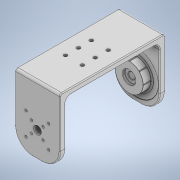
# Autodesk Inventor part: мотор_плеча_2_v2
Saved by Autodesk Inventor 2022 (Build 260153000, 153)
## iProperties
Created: 2022-12-04
Part Number: мотор_плеча_2_v2
Material: Типовые
Document SubType Name: Modeling
Designer: Папа
Density: 1 g/cm^3
Appearance: По умолчанию
Author: Папа
Autodesk Inventor part; units mm, degrees
ref_plane "YZ Plane" through (0, 0, 0) normal (1, 0, 0) x (0, 1, 0)
ref_plane "XZ Plane" through (0, 0, 0) normal (0, 1, 0) x (-1, 0, 0)
ref_plane "XY Plane" through (0, 0, 0) normal (0, 0, 1) x (1, 0, 0)
sketch "Эскиз1" plane through (0, 0, 0) normal (0, 1, 0) x (-1, 0, 0)
  line L0 (-20, -46.7) -> (20, -46.7)
  line L1 (20, -46.7) -> (20, 46.7)
  line L2 (20, 46.7) -> (-20, 46.7)
  line L3 (-20, 46.7) -> (-20, -46.7)
  line L4 (-20, -46.7) -> (20, 46.7) construction
  line L5 (20, -46.7) -> (-20, 46.7) construction
  point P0 (0, 0)
  dimension "d0" = 40
  dimension "d1" = 93.4
  constraints: 12 end point, 2 midpoint, 2 parallel, 1 horizontal, 1 perpendicular
  measures "d0" distance between parallel lines of L3 L1
  measures "d1" distance of L0.end L1.end
extrude "Выдавливание1" add sketch "Эскиз1" along normal blind 5
sketch "Эскиз5" plane through (0, 0, 0) normal (0, -1, 0) x (1, 0, 0)
  line L0 (22.9, 22.9) -> (22.9, -22.9)
  line L1 (22.9, -22.9) -> (-22.9, -22.9)
  line L2 (-22.9, -22.9) -> (-22.9, 22.9)
  line L3 (-22.9, 22.9) -> (22.9, 22.9)
  circle A0 centre (0, 0) radius 12.5
  dimension "d16" = 45.8
  dimension "d17" = 25
  constraints: 8 end point, 2 coincident, 1 centre point, 1 horizontal, 9 other
  measures "d16" distance of L2.end L0.start
  measures "d17" diameter of A0
extrude "Выдавливание5" [suppressed]
fillet "Сопряжение3" [suppressed]
ref_plane "РабПлоскость1" through (20, 0, 0) normal (0, 0, -1) x (-1, 0, 0)
sketch "Эскиз6" plane through (-20, 0, 46.7) normal (0, 0, 1) x (1, 0, 0)
  line L0 (40, 5) -> (42.9, 5) projected
  line L1 (40, 5) -> (0, 5)
  line L2 (0, 5) -> (0, -55)
  line L3 (0, -55) -> (40, -55)
  line L4 (40, -55) -> (40, 5)
  line L5 (0, 0) -> (40, 0) projected
  point P0 (20, 0)
  dimension "d25" = 55
  constraints: 8 end point, 2 parallel, 1 horizontal, 1 perpendicular, 1 point on line
  measures "d25" distance between parallel lines of L5 L3
extrude "Выдавливание6" add sketch "Эскиз6" against normal blind 5 contours L4 L3 L2 L5
fillet "Сопряжение4" radius 5 1 edges at (0, 0, 41.7)
fillet "Сопряжение5" radius 16 2 edges at (-20, -55, 44.2) (20, -55, 44.2)
mirror "Зеркальное отражение2" about plane through (20, 0, 0) normal (0, 0, -1) of "Выдавливание6", "Сопряжение5", "Сопряжение4"
sketch "Эскиз7" plane through (-20, 0, 41.7) normal (0, 0, -1) x (-1, 0, 0)
  line L0 (-40, -39) -> (-40, 5) projected
  line L1 (0, -39) -> (0, 5) projected
  line L2 (0, -10) -> (-40, -10)
  line L3 (-40, -10) -> (-40, -55)
  line L4 (-40, -55) -> (0, -55)
  line L5 (0, -55) -> (0, -10)
  line L6 (-24, -55) -> (-16, -55) projected
  arc A0 (-40, -39) -> (-24, -55) centre (-24, -39) ccw projected
  line L7 (-24, -55) -> (-16, -55) projected
  arc A1 (-16, -55) -> (0, -39) centre (-16, -39) ccw projected
  line L8 (0, -39) -> (0, -5) projected
  line L9 (-40, -5) -> (0, -5) projected
  line L10 (-40, -5) -> (-40, -39) projected
  circle A2 centre (-20, -32.5) radius 3.5
  line L11 (-40, -5) -> (-40, -39) projected
  line L12 (0, -10) -> (-40, -10)
  line L13 (-40, -10) -> (-40, -5)
  line L14 (-40, -5) -> (0, -5)
  line L15 (0, -5) -> (0, -10)
  line L16 (0, -55) -> (-40, -10) construction
  point P0 (-20, 0)
  dimension "d31" = 40
  dimension "d33" = 7
  dimension "d107" = 5
  constraints: 18 end point, 4 parallel, 2 horizontal, 2 midpoint, 2 perpendicular, 1 centre point, 1 collinear, 1 point on line
  measures "d31" distance of L3.end L4.end
  measures "d33" diameter of A2
  measures "d107" distance between parallel lines of L14 L2
extrude "Выдавливание7" cut sketch "Эскиз7" against normal up to surface (5 mm away) contours A2
sketch "Эскиз8" plane through (-20, -5, -41.7) normal (0, 0, 1) x (1, 0, 0)
  line L0 (40, 0) -> (40, -50)
  line L1 (40, -50) -> (0, -50)
  line L2 (0, -50) -> (0, 0)
  line L3 (24, -50) -> (16, -50) projected
  line L4 (40, 0) -> (40, -34) projected
  circle A0 centre (20, -27.5) radius 18.9
  circle A1 centre (20, -27.5) radius 14.5
  line L5 (0, 0) -> (40, 0) projected
  line L6 (0, 0) -> (40, 0)
  line L7 (40, 0) -> (40, -5)
  line L8 (40, -5) -> (0, -5)
  line L9 (0, -5) -> (0, 0)
  point P0 (20, 5)
  dimension "d36" = 37.8
  dimension "d108" = 5
  dimension "d120" = 29
  constraints: 14 end point, 3 parallel, 2 centre point, 2 coincident, 2 collinear, 1 horizontal, 1 perpendicular, 1 point on line
  measures "d36" diameter of A0
  measures "d108" distance between parallel lines of L8 L5
  measures "d120" diameter of A1
extrude "Выдавливание8" cut sketch "Эскиз8" against normal blind 0.2 contours A0
sketch "Эскиз9" plane through (0, -32.5, -41.7) normal (0, 0, 1) x (1, 0, 0)
  circle A0 centre (0, 0) radius 18.9 projected
  circle A1 centre (0, 0) radius 12.35
  point P0 (0, 32.5)
  dimension "d40" = 24.7
  constraints: 1 centre point, 1 coincident
  measures "d40" diameter of A1
extrude "Выдавливание9" add sketch "Эскиз9" along normal blind 6.9 contours A1
sketch "Эскиз10" plane through (0, -32.5, -34.8) normal (0, 0, 1) x (1, 0, 0)
  circle A0 centre (0, 0) radius 12.35 projected
  circle A1 centre (-12.35, 0) radius 0.25
  point P0 (0, 32.5)
  point P1 (-12.3475, -0.25)
  point P2 (-12.3475, 0.25)
  dimension "d44" = 0.5
  constraints: 1 centre point, 2 other
  measures "d44" diameter of A1
extrude "Выдавливание10" add sketch "Эскиз10" against normal up to surface (6.9 mm away) contours A0 A1 picked at (-12.4325, 0.0101)
fillet "Сопряжение7" radius 0.4 2 edges at (-12.3475, -32.25, -38.25) (-12.3475, -32.75, -38.25)
pattern_circular "Круговой массив1" count 8 over 360 about axis through (0, -32.5, -41.7) along (0, 0, 1) of "Сопряжение7", "Выдавливание10"
fillet "Сопряжение8" radius 0.2 66 edges at (-8.9941, -41.0216, -34.8) (-8.9095, -41.4095, -34.8) (-8.5216, -41.4941, -34.8) (-4.7261, -43.9099, -34.8) (-0.3341, -44.8854, -34.8) (0, -45.1, -34.8) (0.3341, -44.8854, -34.8) (4.7261, -43.9099, -34.8) (8.5216, -41.4941, -34.8) (8.9095, -41.4095, -34.8) (8.9941, -41.0216, -34.8) (11.4099, -37.2261, -34.8) (12.3854, -32.8341, -34.8) (12.6, -32.5, -34.8) (12.3854, -32.1659, -34.8) (11.4099, -27.7739, -34.8) (8.9941, -23.9784, -34.8) (8.9095, -23.5905, -34.8) (8.5216, -23.5059, -34.8) (4.7261, -21.0901, -34.8) (0.3341, -20.1146, -34.8) (0, -19.9, -34.8) (-0.3341, -20.1146, -34.8) (-4.7261, -21.0901, -34.8) (-8.5216, -23.5059, -34.8) (-8.9095, -23.5905, -34.8) (-8.9941, -23.9784, -34.8) (-11.4099, -27.7739, -34.8) (-12.3854, -32.1659, -34.8) (-12.6, -32.5, -34.8) (-12.3854, -32.8341, -34.8) (-11.4099, -37.2261, -34.8) (-12.3854, -32.8341, -41.7) (-12.6, -32.5, -41.7) (-12.3854, -32.1659, -41.7) (-11.4099, -27.7739, -41.7) (-8.9941, -23.9784, -41.7) (-8.9095, -23.5905, -41.7) (-8.5216, -23.5059, -41.7) (-4.7261, -21.0901, -41.7) (-0.3341, -20.1146, -41.7) (0, -19.9, -41.7) (0.3341, -20.1146, -41.7) (4.7261, -21.0901, -41.7) (8.5216, -23.5059, -41.7) (8.9095, -23.5905, -41.7) (8.9941, -23.9784, -41.7) (11.4099, -27.7739, -41.7) (12.3854, -32.1659, -41.7) (12.6, -32.5, -41.7) (12.3854, -32.8341, -41.7) (11.4099, -37.2261, -41.7) (8.9941, -41.0216, -41.7) (8.9095, -41.4095, -41.7) (8.5216, -41.4941, -41.7) (4.7261, -43.9099, -41.7) (0.3341, -44.8854, -41.7) (0, -45.1, -41.7) (-0.3341, -44.8854, -41.7) (-4.7261, -43.9099, -41.7) (-8.5216, -41.4941, -41.7) (-8.9095, -41.4095, -41.7) (-8.9941, -41.0216, -41.7) (-11.4099, -37.2261, -41.7) (-18.9, -32.5, -41.7) (-18.9, -32.5, -41.9)
fillet "Сопряжение11" radius 2 2 edges at (0, 5, -46.7) (0, 5, 46.7)
ref_plane "РабПлоскость3" through (3.7349, -5, -34.5) normal (0, 0, 1) x (1, 0, 0)
sketch "Эскиз17" plane through (-20, -5, -41.7) normal (0, 0, 1) x (1, 0, 0)
  circle A0 centre (20, -27.5) radius 14.5 projected
  circle A1 centre (20, -27.5) radius 20.9
  circle A2 centre (20, -27.5) radius 22.9
  point P0 (20, 5)
  point P1 (0, -21.4329)
  point P2 (40, -21.4329)
  dimension "d70" = 2
  constraints: 2 coincident, 1 centre point, 4 other
extrude "Выдавливание14" [suppressed]
fillet "Сопряжение14" radius 0.8 32 edges at (-20, -22, -41.7) (0, -55, -41.7) (-15.3137, -50.3137, -41.7) (0, -55, -46.7) (-20, -18, -46.7) (-15.3137, -50.3137, -46.7) (15.3137, -50.3137, -41.7) (20, -22, -41.7) (15.3137, -50.3137, -46.7) (20, -18, -46.7) (20, -1.4645, -40.2355) (20, 0, 0) (-20, -1.4645, -40.2355) (-20, 0, 0) (20, 4.4142, -46.1142) (20, 5, 0) (-20, 4.4142, -46.1142) (-20, 5, 0) (20, 4.4142, 46.1142) (20, -18, 46.7) (15.3137, -50.3137, 46.7) (0, -55, 46.7) (-15.3137, -50.3137, 46.7) (-20, -18, 46.7) (-20, 4.4142, 46.1142) (20, -1.4645, 40.2355) (20, -22, 41.7) (15.3137, -50.3137, 41.7) (0, -55, 41.7) (-15.3137, -50.3137, 41.7) (-20, -22, 41.7) (-20, -1.4645, 40.2355)
sketch "Эскиз19" plane through (0, -32.5, -34.8) normal (0, 0, 1) x (1, 0, 0)
  circle A0 centre (0, 0) radius 5.75
  arc A1 (8.5045, 9.229) -> (0.5123, 12.5395) centre (0, 0) ccw projected
  point P0 (0, 32.5)
  dimension "d79" = 11.5
  constraints: 1 centre point, 1 coincident
  measures "d79" diameter of A0
extrude "Выдавливание16" cut sketch "Эскиз19" against normal blind 2
sketch "Эскиз20" plane through (0, -32.5, -36.8) normal (0, 0, 1) x (1, 0, 0)
  circle A0 centre (0, 0) radius 3
  circle A1 centre (0, 0) radius 5.75 projected
  point P0 (0, 32.5)
  dimension "d82" = 6
  constraints: 1 centre point, 1 concentric
  measures "d82" diameter of A0
extrude "Выдавливание17" cut sketch "Эскиз20" against normal blind 0.5 contours A0
fillet "Сопряжение16" radius 0.3 4 edges at (-5.75, -32.5, -34.8) (-5.75, -32.5, -36.8) (-3, -32.5, -37.3) (-3, -32.5, -36.8)
sketch "Эскиз21" plane through (0, 5, 0) normal (0, 1, 0) x (1, 0, 0)
  line L0 (7.5, -14.3) -> (-7.5, -14.3) construction
  line L1 (-7.5, -14.3) -> (-7.5, 8.7) construction
  line L2 (-7.5, 8.7) -> (7.5, 8.7) construction
  line L3 (7.5, 8.7) -> (7.5, -14.3) construction
  line L4 (7.5, -14.3) -> (-7.5, 8.7) construction
  line L5 (-7.5, -14.3) -> (7.5, 8.7) construction
  circle A0 centre (-7.5, -14.3) radius 1.55
  circle A1 centre (-7.5, -2.8) radius 1.55
  circle A2 centre (-7.5, 8.7) radius 1.55
  circle A3 centre (7.5, -14.3) radius 1.55
  circle A4 centre (7.5, -2.8) radius 1.55
  circle A5 centre (7.5, 8.7) radius 1.55
  line L6 (19.2, 44.7) -> (19.2, -44.7) construction
  line L7 (-19.2, 44.7) -> (19.2, 44.7) construction
  line L8 (-19.2, -44.7) -> (-19.2, 44.7) construction
  line L9 (19.2, -44.7) -> (-19.2, -44.7) construction
  line L10 (19.2, -44.7) -> (-19.2, -44.7) construction
  line L11 (-19.2, 44.7) -> (19.2, -44.7) construction
  line L12 (-19.2, 44.7) -> (19.2, 44.7) construction
  line L13 (19.2, 44.7) -> (-19.2, -44.7) construction
  line L14 (0, 44.7) -> (0, -2.8) construction
  line L15 (19.2, 0) -> (0, 0) construction
  point P0 (-22.7, -22.7739)
  point P1 (-22.7, 22.7739)
  point P2 (22.9, 22.9)
  dimension "d86" = 15
  dimension "d87" = 23
  dimension "d88" = 3.1
  dimension "d91" = 11.5
  dimension "d94" = 15
  dimension "d121" = 2.8
  constraints: 20 end point, 6 centre point, 5 midpoint, 2 horizontal, 2 parallel, 2 vertical, 1 coincident, 1 perpendicular, 1 point on line, 10 other
  measures "d86" distance of L1.end L2.end
  measures "d87" distance of L0.end L1.end
  measures "d88" diameter of A0
  measures "d91" distance of A0.centre A1.centre
  measures "d94" distance of A0.centre A3.centre
  measures "d121" distance from line of L14.end L15
extrude "Выдавливание18" cut sketch "Эскиз21" against normal blind 10
chamfer "Фаска2" distance 1.8 angle 45 6 edges at (5.95, 0, 14.3) (5.95, 0, 2.8) (5.95, 0, -8.7) (-9.05, 0, -8.7) (-9.05, 0, 2.8) (-9.05, 0, 14.3) measured on face at (-9.55, 0, -8.7) measured on face at (-9.55, 0, 2.8) measured on face at (5.45, 0, -8.7) measured on face at (-9.55, 0, 14.3) measured on face at (5.45, 0, 2.8) measured on face at (5.45, 0, 14.3)
ref_plane "РабПлоскость4" through (0, -21.3461, -46.5) normal (1, 0, 0) x (0, 0, -1)
sketch "Эскиз22" plane through (0, -21.3461, -46.5) normal (1, 0, 0) x (0, 0, -1)
  line L0 (-11.5, -23.7539) -> (-5, -23.7539) projected
  line L1 (-11.7, -23.2938) -> (-11.7, -20.0888) projected
  line L2 (-11.1, -23.1539) -> (-11.7, -23.1539) construction
  line L3 (-11.7, -23.1539) -> (-11.7, -23.7539)
  line L4 (-11.7, -23.7539) -> (-11.1, -23.7539)
  line L5 (-11.1, -23.7539) -> (-11.1, -23.1539) construction
  line L6 (-11.7, -23.1539) -> (-11.1, -23.7539)
  line L7 (18.88, -11.1539) -> (-111.88, -11.1539) projected
  point P0 (-46.5, 21.3461)
  point P1 (-11.7, -23.1539)
  point P2 (-11.7, -23.2938)
  point P3 (-11.5, -23.7539)
  dimension "d109" = 0.6
  constraints: 10 end point, 2 collinear, 2 parallel, 2 perpendicular, 1 horizontal
  measures "d109" distance of L4.end L2.start
revolve "Вращение1" [suppressed]
sketch "Эскиз23" plane through (-20, 0, 41.7) normal (0, 0, -1) x (-1, 0, 0)
  circle A0 centre (-20, -32.5) radius 3.5 construction
  circle A1 centre (-20, -32.5) radius 5.1265 construction
  line L0 (-25.1265, -37.6265) -> (-14.8735, -37.6265) construction
  line L1 (-14.8735, -37.6265) -> (-14.8735, -27.3735) construction
  line L2 (-14.8735, -27.3735) -> (-25.1265, -27.3735) construction
  line L3 (-25.1265, -27.3735) -> (-25.1265, -37.6265) construction
  circle A2 centre (-25.1265, -27.3735) radius 1.05
  circle A3 centre (-14.8735, -27.3735) radius 1.05
  circle A4 centre (-14.8735, -37.6265) radius 1.05
  circle A5 centre (-25.1265, -37.6265) radius 1.05
  line L4 (-30.0763, -42.5763) -> (-9.9237, -42.5763) construction
  line L5 (-9.9237, -42.5763) -> (-9.9237, -22.4237) construction
  line L6 (-9.9237, -22.4237) -> (-30.0763, -22.4237) construction
  line L7 (-30.0763, -22.4237) -> (-30.0763, -42.5763) construction
  circle A6 centre (-30.0763, -22.4237) radius 1.05
  circle A7 centre (-30.0763, -42.5763) radius 1.05
  circle A8 centre (-9.9237, -42.5763) radius 1.05
  circle A9 centre (-9.9237, -22.4237) radius 1.05
  point P0 (-20, 0)
  dimension "d111" = 7.25
  dimension "d112" = 2.1
  dimension "d113" = 7
  dimension "d116" = 7
  dimension "d117" = 7
  constraints: 16 end point, 9 centre point, 9 coincident, 7 equal radius, 4 parallel, 4 tangent, 3 perpendicular, 2 horizontal
  measures "d111" distance of A1.centre L2.end
  measures "d112" diameter of A2
  measures "d113" distance of L6.end L2.end
  measures "d116" distance of L5.end L1.end
  measures "d117" distance of L4.end L0.end
extrude "Выдавливание19" cut sketch "Эскиз23" against normal blind 10
